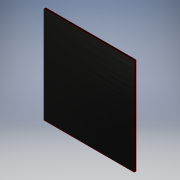
# Autodesk Inventor part: Front PC Cover
Saved by Autodesk Inventor 2019.4 (Build 234330000, 330)
## iProperties
Created: 2020-01-23
Part Number: Front PC Cover
Material: Polycarbonate, Smoke
Document SubType Name: Modeling
Designer: admin
Density: 1.2 g/cm^3
Appearance: Red
Author: admin
Autodesk Inventor part; units mm, degrees
ref_plane "YZ Plane" through (0, 0, 0) normal (1, 0, 0) x (0, 1, 0)
ref_plane "XZ Plane" through (0, 0, 0) normal (0, 1, 0) x (-1, 0, 0)
ref_plane "XY Plane" through (0, 0, 0) normal (0, 0, 1) x (1, 0, 0)
sketch "Sketch1" plane through (0, 0, 0) normal (0, 0, 1) x (1, 0, 0)
  line L0 (-119, -127.5) -> (119, -127.5)
  line L1 (119, -127.5) -> (119, 127.5)
  line L2 (119, 127.5) -> (-119, 127.5)
  line L3 (-119, 127.5) -> (-119, -127.5)
  line L4 (-119, -127.5) -> (119, 127.5) construction
  line L5 (119, -127.5) -> (-119, 127.5) construction
  point P0 (0, 0)
  dimension "d0" = 238
  dimension "d1" = 255
  constraints: 12 end point, 2 midpoint, 2 parallel, 1 horizontal, 1 perpendicular
  measures "d0" distance of L1.end L2.end
  measures "d1" distance of L0.end L1.end
extrude "Extrusion1" add sketch "Sketch1" against normal blind 5
body "Solid1"
